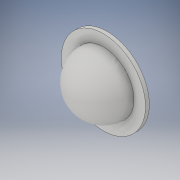
# Autodesk Inventor part: DomeTest
Saved by Autodesk Inventor 2018 (Build 220112000, 112)
## iProperties
Created: 2019-02-18
Part Number: DomeTest
Material: Generic
Document SubType Name: Modeling
Designer: anirudh
Density: 1 g/cm^3
Appearance: Default
Author: anirudh
Autodesk Inventor part; units mm, degrees
ref_plane "YZ Plane" through (0, 0, 0) normal (1, 0, 0) x (0, 1, 0)
ref_plane "XZ Plane" through (0, 0, 0) normal (0, 1, 0) x (-1, 0, 0)
ref_plane "XY Plane" through (0, 0, 0) normal (0, 0, 1) x (1, 0, 0)
sketch "Sketch1" plane through (0, 0, 0) normal (0, 0, 1) x (1, 0, 0)
  line L0 (0, 0) -> (0, 50.8)
  arc A0 (0, 50.8) -> (0, 0) centre (0, 25.4) ccw
  line L1 (0, 0) -> (0, -13.8056)
  dimension "d0" = 50.8
  constraints: 4 end point, 2 point on circle, 2 vertical, 1 centre point, 1 midpoint
  measures "d0" distance of L0.start L0.end
revolve "Revolution1" add sketch "Sketch1" angle 180 about axis through (0, 0, 0) along (0, 1, 0)
sketch "Sketch2" plane through (0, 25.4, 0) normal (0, 0, -1) x (-1, 0, 0)
  circle A0 centre (0, 0) radius 34.925
  point P0 (0, -25.4)
  dimension "d2" = 69.85
  constraints: 1 centre point
  measures "d2" diameter of A0
extrude "Extrusion1" add sketch "Sketch2" along normal blind 3.175
body "Solid1"
